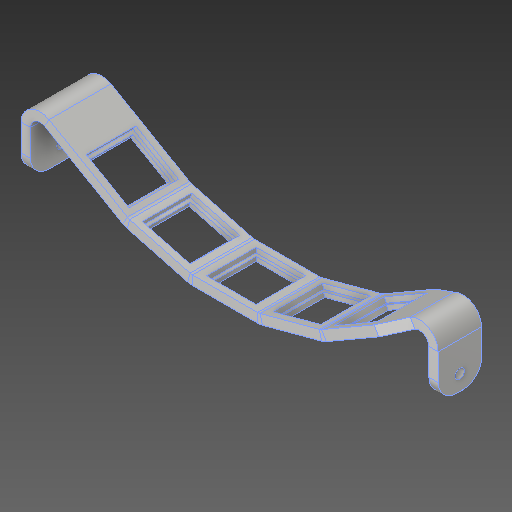
# Autodesk Inventor part: keyplate5
Saved by Autodesk Inventor 2018 (Build 220112000, 112)
## iProperties
Created: 2018-05-25
Part Number: keyplate5
Material: アルミニウム 6061
Document SubType Name: Sheet Metal
Designer: NaMACHAN
Density: 2.7 g/cm^3
Sheet Metal Rule: Al2mm
Appearance: アルミニウム - フラット
Mass: 16.9543 g
Surface Area: 65.7623 cm^2
Volume: 6.27936 cm^3
Author: NaMACHAN
Autodesk Inventor part; units mm, degrees
ref_plane "YZ Plane" through (0, 0, 0) normal (1, 0, 0) x (0, 1, 0)
ref_plane "XZ Plane" through (0, 0, 0) normal (0, 1, 0) x (-1, 0, 0)
ref_plane "XY Plane" through (0, 0, 0) normal (0, 0, 1) x (1, 0, 0)
sketch "スケッチ1" plane through (0, 0, 0) normal (0, 1, 0) x (-1, 0, 0)
  line L0 (-10.5, -10) -> (10.5, -10)
  line L1 (10.5, -10) -> (10.5, 10)
  line L2 (10.5, 10) -> (-10.5, 10)
  line L3 (-10.5, 10) -> (-10.5, -10)
  line L4 (-10.5, -10) -> (10.5, 10) construction
  line L5 (10.5, -10) -> (-10.5, 10) construction
  line L6 (-7, -7) -> (7, -7)
  line L7 (7, -7) -> (7, 7)
  line L8 (7, 7) -> (-7, 7)
  line L9 (-7, 7) -> (-7, -7)
  line L10 (-7, -7) -> (7, 7) construction
  line L11 (7, -7) -> (-7, 7) construction
  point P0 (0, 0)
  dimension "d0" = 21
  dimension "d1" = 20
  dimension "d2" = 14
  dimension "d3" = 14
  measures "d0" distance of L2.end L1.end
  measures "d1" distance of L1.end L0.end
  measures "d2" distance of L8.end L7.end
  measures "d3" distance of L7.end L6.end
extrude "プレート1" add sketch "スケッチ1" along normal blind 3
sketch "スケッチ2" plane through (-11.2765, 3.1022, 10) normal (-0.258819, -0.9659258, 0) x (0.9659258, -0.258819, 0)
  line L0 (0, -20) -> (0, 0)
  line L1 (0, 0) -> (-20.2101, 0)
  line L2 (-20.2101, 0) -> (-20.2101, -20)
  line L3 (-20.2101, -20) -> (0, -20)
  constraints: 6 end point, 1 horizontal, 1 perpendicular, 1 vertical
edge flange "フランジ1" height 21 angle 15 thickness 3 bend radius 3 thickness toward (-0.258819, -0.9659258, 0) relief straight relief width 3 relief depth 1.5 edges at (-10.5, 3, 0) wall of the first edge with corners at (-11.2765, 3.1022, -10) (-11.2765, 3.1022, 10) (-30.7979, 8.333, 10) (-30.7979, 8.333, -10)
bend "曲げ1"
corner "コーナー1"
sketch "スケッチ3" plane through (11.2765, 3.1022, -10) normal (0.258819, -0.9659258, 0) x (0.9659258, 0.258819, 0)
  line L0 (0, 20) -> (0, 0)
  line L1 (0, 0) -> (20.2101, 0)
  line L2 (20.2101, 0) -> (20.2101, 20)
  line L3 (20.2101, 20) -> (0, 20)
  constraints: 8 end point
edge flange "フランジ2" height 21 angle 15 thickness 3 bend radius 3 thickness toward (0.258819, -0.9659258, 0) relief straight relief width 3 relief depth 1.5 edges at (10.5, 3, 0) wall of the first edge with corners at (11.2765, 3.1022, 10) (11.2765, 3.1022, -10) (30.7979, 8.333, -10) (30.7979, 8.333, 10)
bend "曲げ2"
corner "コーナー2"
sketch "スケッチ6" plane through (-31.5214, 8.6327, 10) normal (-0.5, -0.8660254, 0) x (0.8660254, -0.5, 0)
  line L0 (0, -20) -> (0, 0)
  line L1 (0, 0) -> (-29.2101, 0)
  line L2 (-29.2101, 0) -> (-29.2101, -20)
  line L3 (-29.2101, -20) -> (0, -20)
  constraints: 6 end point, 1 horizontal, 1 perpendicular, 1 vertical
edge flange "フランジ5" height 30 angle 15 thickness 3 bend radius 3 thickness toward (-0.5, -0.8660254, 0) relief straight relief width 3 relief depth 1.5 edges at (-30.7979, 8.333, 0) wall of the first edge with corners at (-31.5214, 8.6327, -10) (-31.5214, 8.6327, 10) (-56.8181, 23.2377, 10) (-56.8181, 23.2377, -10)
bend "曲げ5"
corner "コーナー5"
sketch "スケッチ7" plane through (11.2765, 3.1022, 10) normal (-0.258819, 0.9659258, 0) x (0.9659258, 0.258819, 0)
  line L0 (3.2367, 17) -> (17.2367, 17)
  line L1 (17.2367, 17) -> (17.2367, 3)
  line L2 (17.2367, 3) -> (3.2367, 3)
  line L3 (3.2367, 3) -> (3.2367, 17)
  line L4 (3.2367, 17) -> (17.2367, 3) construction
  line L5 (17.2367, 17) -> (3.2367, 3) construction
  line L6 (20.2101, 0) -> (0, 0) projected
  line L7 (-0.7765, 20) -> (-0.7765, 0) projected
  point P0 (-11.6951, 10)
  point P1 (10.2367, 10)
  point P2 (10.2367, 10)
  point P3 (10.2367, 0)
  point P4 (20.4734, 0)
  point P5 (10.2367, 10)
  point P6 (-0.7765, 10)
  dimension "d55" = 14
  dimension "d56" = 14
  constraints: 12 end point, 5 midpoint, 2 parallel, 1 horizontal, 1 horizontal alignment, 1 perpendicular, 1 point on line, 1 vertical alignment
  measures "d55" distance of L1.end L2.end
  measures "d56" distance of L0.end L1.end
extrude "押し出し1" cut sketch "スケッチ7" against normal blind 10
sketch "スケッチ9" plane through (-11.2765, 3.1022, 10) normal (0.258819, 0.9659258, 0) x (0.9659258, -0.258819, 0)
  line L0 (-17.105, 17) -> (-3.105, 17)
  line L1 (-3.105, 17) -> (-3.105, 3)
  line L2 (-3.105, 3) -> (-17.105, 3)
  line L3 (-17.105, 3) -> (-17.105, 17)
  line L4 (-17.105, 17) -> (-3.105, 3) construction
  line L5 (-3.105, 17) -> (-17.105, 3) construction
  line L6 (-20.2101, 20) -> (-20.2101, 0) projected
  line L7 (-20.2101, 0) -> (0, 0) projected
  point P0 (11.6951, 10)
  point P1 (-10.105, 10)
  point P2 (-10.105, 10)
  point P3 (-20.2101, 10)
  point P4 (-10.105, 10)
  point P5 (-10.105, 0)
  dimension "d63" = 14
  dimension "d64" = 14
  constraints: 12 end point, 6 midpoint, 2 parallel, 1 horizontal, 1 horizontal alignment, 1 perpendicular, 1 vertical alignment
  measures "d63" distance of L1.end L2.end
  measures "d64" distance of L0.end L1.end
extrude "押し出し3" cut sketch "スケッチ9" against normal blind 10
sketch "スケッチ15" plane through (-31.5214, 8.6327, 10) normal (0.5, 0.8660254, 0) x (0.8660254, -0.5, 0)
  line L0 (-2.7008, 17) -> (-16.7008, 17)
  line L1 (-16.7008, 17) -> (-16.7008, 3)
  line L2 (-16.7008, 3) -> (-2.7008, 3)
  line L3 (-2.7008, 3) -> (-2.7008, 17)
  line L4 (-2.7008, 17) -> (-16.7008, 3) construction
  line L5 (-16.7008, 17) -> (-2.7008, 3) construction
  line L6 (0.7765, 20) -> (0.7765, 0) projected
  line L7 (-29.2101, 20) -> (0, 20) projected
  point P0 (31.6147, 10)
  point P1 (-9.7008, 10)
  point P2 (-9.7008, 10)
  point P3 (0.7765, 10)
  point P4 (-9.7008, 10)
  point P5 (-9.7008, 20)
  point P6 (-19.4016, 20)
  dimension "d93" = 14
  dimension "d94" = 14
  constraints: 12 end point, 5 midpoint, 2 parallel, 1 horizontal, 1 horizontal alignment, 1 perpendicular, 1 point on line, 1 vertical alignment
  measures "d93" distance of L2.end L1.end
  measures "d94" distance of L1.end L0.end
extrude "押し出し8" cut sketch "スケッチ15" against normal blind 10
sketch "スケッチ28" plane through (-62.8181, 18.0416, -10) normal (-1, 0, 0) x (0, -1, 0)
  line L0 (0, 20) -> (0, 0)
  line L1 (0, 0) -> (14.6077, 0)
  line L2 (14.6077, 0) -> (14.6077, 20)
  line L3 (14.6077, 20) -> (0, 20)
  constraints: 6 end point, 1 horizontal, 1 perpendicular, 1 vertical
edge flange "フランジ13" height 25 angle 120 thickness 3 bend radius 3 thickness toward (-1, 0, 0) relief straight relief width 3 relief depth 1.5 edges at (-58.3181, 20.6396, 0) wall of the first edge with corners at (-62.8181, 18.0416, 10) (-62.8181, 18.0416, -10) (-62.8181, 3.4339, -10) (-62.8181, 3.4339, 10)
bend "曲げ13"
corner "コーナー13"
ref_plane "作業平面1" through (30.7979, 8.333, 10) normal (-0.5, 0.8660254, 0) x (0, 0, -1)
sketch "スケッチ31" plane through (30.7979, 8.333, 10) normal (-0.5, 0.8660254, 0) x (0, 0, -1)
  line L0 (0, 0) -> (0, -20)
  line L1 (0, -20) -> (3, -30)
  line L2 (3, -30) -> (17, -30)
  line L3 (17, -30) -> (20, -20)
  line L4 (20, 0) -> (20, 19.5214)
  line L5 (20, -20) -> (20, 0)
  line L6 (0, 0) -> (20, 0)
  point P0 (10, 30.8383)
  point P1 (10, -30)
  point P2 (10, 0)
  dimension "d220" = 20
  dimension "d221" = 30
  dimension "d222" = 14
  measures "d220" distance of L0.start L0.end
  measures "d221" distance between parallel lines of L6 L2
  measures "d222" distance of L1.end L2.end
sheet face with bend "面2" sketch "スケッチ31" thickness 3 toward (0.5, -0.8660254, 0) bend radius 3 relief straight relief width 3 relief depth 1.5
bend "曲げ15"
sketch "スケッチ32" plane through (30.7979, 8.333, 10) normal (-0.5, 0.8660254, 0) x (0.8660254, 0.5, 0)
  line L0 (3.895, 3) -> (17.895, 3)
  line L1 (17.895, 3) -> (17.895, 17)
  line L2 (17.895, 17) -> (3.895, 17)
  line L3 (3.895, 17) -> (3.895, 3)
  line L4 (3.895, 3) -> (17.895, 17) construction
  line L5 (17.895, 3) -> (3.895, 17) construction
  line L6 (-0.3815, 0) -> (-0.3815, 20) projected
  line L7 (0.395, 0) -> (0.395, 20) projected
  point P0 (-30.8383, 10)
  point P1 (10.895, 10)
  point P2 (10.895, 10)
  point P3 (-0.3815, 10)
  dimension "d228" = 14
  dimension "d229" = 14
  dimension "d230" = 10.5
  constraints: 12 end point, 4 midpoint, 2 parallel, 1 horizontal, 1 horizontal alignment, 1 perpendicular
  measures "d228" distance of L2.end L1.end
  measures "d229" distance of L1.end L0.end
  measures "d230" distance from line of L7 point (10.895, 10)
extrude "押し出し13" cut sketch "スケッチ32" against normal blind 10
sketch "スケッチ33" plane through (62.7787, 18.1368, 7) normal (1, 0, 0) x (0, 1, 0)
  line L0 (0, -14) -> (0, 0)
  line L1 (0, 0) -> (-14.6077, 0)
  line L2 (-14.6077, 0) -> (-14.6077, -14)
  line L3 (-14.6077, -14) -> (0, -14)
  constraints: 6 end point, 1 horizontal, 1 perpendicular, 1 vertical
edge flange "フランジ15" height 25 angle 120 thickness 3 bend radius 3 thickness toward (1, 0, 0) relief straight relief width 3 relief depth 1.5 edges at (58.2787, 20.7349, 0) wall of the first edge with corners at (62.7787, 18.1368, -7) (62.7787, 18.1368, 7) (62.7787, 3.5291, 7) (62.7787, 3.5291, -7)
bend "曲げ16"
corner "コーナー15"
sketch "スケッチ34" plane through (65.7787, 3.5291, 7) normal (1, 0, 0) x (0, 0, -1)
  line L0 (14, 0) -> (0, 0) projected
  point P0 (7, -3.5291)
  point P1 (7, 5)
  dimension "d243" = 5
  constraints: 1 vertical alignment
  measures "d243" distance from line of L0 point (7, 5)
hole "穴3" at (65.7787, 8.5291, 0) direction (-1, 0, 0) diameter 3 depth 3 tip angle 118
sketch "スケッチ35" plane through (-65.8181, 3.4339, -10) normal (-1, 0, 0) x (0, 0, 1)
  circle A0 centre (10, 5.0953) radius 1.5 projected
  point P0 (10, -3.4339)
  constraints: 1 coincident
hole "穴4" at (-65.8181, 8.5291, 0) direction (1, 0, 0) diameter 3 depth 3 tip angle 118
sketch "スケッチ36" plane through (-31.5214, 8.6327, 10) normal (0.5, 0.8660254, 0) x (0.8660254, -0.5, 0)
  line L0 (-1.7008, 18) -> (-17.7008, 18)
  line L1 (-17.7008, 18) -> (-17.7008, 2)
  line L2 (-17.7008, 2) -> (-1.7008, 2)
  line L3 (-1.7008, 2) -> (-1.7008, 18)
  line L4 (-1.7008, 18) -> (-17.7008, 2) construction
  line L5 (-17.7008, 18) -> (-1.7008, 2) construction
  line L6 (-16.7008, 3) -> (-16.7008, 17) projected
  line L7 (-16.7008, 17) -> (-2.7008, 17) projected
  point P0 (31.6147, 10)
  point P1 (-9.7008, 10)
  point P2 (-9.7008, 10)
  point P3 (-16.7008, 10)
  point P4 (-9.7008, 10)
  point P5 (-9.7008, 17)
  dimension "d258" = 16
  dimension "d259" = 16
  constraints: 12 end point, 6 midpoint, 2 parallel, 1 horizontal, 1 horizontal alignment, 1 perpendicular, 1 vertical alignment
  measures "d258" distance of L2.end L1.end
  measures "d259" distance of L1.end L0.end
extrude "押し出し14" cut sketch "スケッチ36" against normal blind 1.6
sketch "スケッチ37" plane through (-11.2765, 3.1022, 10) normal (0.258819, 0.9659258, 0) x (0.9659258, -0.258819, 0)
  line L0 (-2.105, 18) -> (-18.105, 18)
  line L1 (-18.105, 18) -> (-18.105, 2)
  line L2 (-18.105, 2) -> (-2.105, 2)
  line L3 (-2.105, 2) -> (-2.105, 18)
  line L4 (-2.105, 18) -> (-18.105, 2) construction
  line L5 (-18.105, 18) -> (-2.105, 2) construction
  line L6 (-17.105, 3) -> (-17.105, 17) projected
  line L7 (-17.105, 17) -> (-3.105, 17) projected
  point P0 (11.6951, 10)
  point P1 (-10.105, 10)
  point P2 (-10.105, 10)
  point P3 (-17.105, 10)
  point P4 (-10.105, 10)
  point P5 (-10.105, 17)
  dimension "d262" = 16
  dimension "d263" = 16
  constraints: 12 end point, 6 midpoint, 2 parallel, 1 horizontal, 1 horizontal alignment, 1 perpendicular, 1 vertical alignment
  measures "d262" distance of L2.end L1.end
  measures "d263" distance of L1.end L0.end
extrude "押し出し15" cut sketch "スケッチ37" against normal blind 1.6
sketch "スケッチ38" plane through (0, 3, 0) normal (0, 1, 0) x (1, 0, 0)
  line L0 (8, 8) -> (-8, 8)
  line L1 (-8, 8) -> (-8, -8)
  line L2 (-8, -8) -> (8, -8)
  line L3 (8, -8) -> (8, 8)
  line L4 (8, 8) -> (-8, -8) construction
  line L5 (-8, 8) -> (8, -8) construction
  point P0 (0, 0)
  dimension "d266" = 16
  dimension "d267" = 16
  constraints: 12 end point, 2 midpoint, 2 parallel, 1 horizontal, 1 perpendicular
  measures "d266" distance of L2.end L1.end
  measures "d267" distance of L1.end L0.end
extrude "押し出し16" cut sketch "スケッチ38" against normal blind 1.6
sketch "スケッチ39" plane through (11.2765, 3.1022, 10) normal (-0.258819, 0.9659258, 0) x (0.9659258, 0.258819, 0)
  line L0 (18.2367, 18) -> (2.2367, 18)
  line L1 (2.2367, 18) -> (2.2367, 2)
  line L2 (2.2367, 2) -> (18.2367, 2)
  line L3 (18.2367, 2) -> (18.2367, 18)
  line L4 (18.2367, 18) -> (2.2367, 2) construction
  line L5 (2.2367, 18) -> (18.2367, 2) construction
  line L6 (3.2367, 3) -> (3.2367, 17) projected
  line L7 (3.2367, 17) -> (17.2367, 17) projected
  point P0 (-11.6951, 10)
  point P1 (10.2367, 10)
  point P2 (10.2367, 10)
  point P3 (3.2367, 10)
  point P4 (10.2367, 10)
  point P5 (10.2367, 17)
  dimension "d270" = 16
  dimension "d271" = 16
  constraints: 12 end point, 6 midpoint, 2 parallel, 1 horizontal, 1 horizontal alignment, 1 perpendicular, 1 vertical alignment
  measures "d270" distance of L2.end L1.end
  measures "d271" distance of L1.end L0.end
extrude "押し出し17" cut sketch "スケッチ39" against normal blind 1.6
sketch "スケッチ40" plane through (30.7979, 8.333, 10) normal (-0.5, 0.8660254, 0) x (0.8660254, 0.5, 0)
  point P0 (-30.8383, 10)
sketch "スケッチ41" plane through (30.7979, 8.333, 10) normal (-0.5, 0.8660254, 0) x (0.8660254, 0.5, 0)
  line L0 (18.895, 18) -> (2.895, 18)
  line L1 (2.895, 18) -> (2.895, 2)
  line L2 (2.895, 2) -> (18.895, 2)
  line L3 (18.895, 2) -> (18.895, 18)
  line L4 (18.895, 18) -> (2.895, 2) construction
  line L5 (2.895, 18) -> (18.895, 2) construction
  line L6 (3.895, 17) -> (17.895, 17) projected
  line L7 (3.895, 3) -> (3.895, 17) projected
  point P0 (-30.8383, 10)
  point P1 (10.895, 10)
  point P2 (10.895, 10)
  point P3 (10.895, 17)
  point P4 (10.895, 10)
  point P5 (3.895, 10)
  dimension "d274" = 16
  dimension "d275" = 16
  constraints: 12 end point, 6 midpoint, 2 parallel, 1 horizontal, 1 horizontal alignment, 1 perpendicular, 1 vertical alignment
  measures "d274" distance of L2.end L1.end
  measures "d275" distance of L1.end L0.end
extrude "押し出し18" cut sketch "スケッチ41" against normal blind 1.6
fillet "コーナーR2" radius 6 4 edges at (64.2787, 3.5291, 7) (64.2787, 3.5291, -7) (-64.3181, 3.4339, 10) (-64.3181, 3.4339, -10)
equation "\"d249\" = Thickness"
equation "\"d256\" = Thickness"
equation "\"d4\" = Thickness"
equation "\"d5\" = BendReliefWidth"
equation "\"d6\" = BendReliefDepth"
equation "\"d7\" = MinimumRemnant"
equation "\"d8\" = TransitionRadius"
equation "\"d11\" = BendRadius"
equation "\"d12\" = CornerReliefSize"
equation "\"d13\" = GapSize"
equation "\"d14\" = JacobiRadiusSize"
equation "\"d15\" = BendReliefWidth"
equation "\"d16\" = BendReliefDepth"
equation "\"d17\" = MinimumRemnant"
equation "\"d18\" = TransitionRadius"
equation "\"d21\" = BendRadius"
equation "\"d22\" = CornerReliefSize"
equation "\"d23\" = GapSize"
equation "\"d24\" = JacobiRadiusSize"
equation "\"d45\" = BendReliefWidth"
equation "\"d46\" = BendReliefDepth"
equation "\"d47\" = MinimumRemnant"
equation "\"d48\" = TransitionRadius"
equation "\"d51\" = BendRadius"
equation "\"d52\" = CornerReliefSize"
equation "\"d53\" = GapSize"
equation "\"d54\" = JacobiRadiusSize"
equation "\"d191\" = BendReliefWidth"
equation "\"d192\" = BendReliefDepth"
equation "\"d193\" = MinimumRemnant"
equation "\"d194\" = TransitionRadius"
equation "\"d197\" = BendRadius"
equation "\"d198\" = CornerReliefSize"
equation "\"d199\" = GapSize"
equation "\"d200\" = JacobiRadiusSize"
equation "\"d223\" = BendRadius"
equation "\"d224\" = BendReliefWidth"
equation "\"d226\" = MinimumRemnant"
equation "\"d225\" = BendReliefDepth"
equation "\"d227\" = TransitionRadius"
equation "\"d233\" = BendReliefWidth"
equation "\"d234\" = BendReliefDepth"
equation "\"d235\" = MinimumRemnant"
equation "\"d236\" = TransitionRadius"
equation "\"d239\" = BendRadius"
equation "\"d240\" = CornerReliefSize"
equation "\"d241\" = GapSize"
equation "\"d242\" = JacobiRadiusSize"
equation "\"BendRadius\" = Thickness"
equation "\"BendReliefWidth\" = Thickness"
equation "\"BendReliefDepth\" = 0.5 * Thickness"
equation "\"CornerReliefSize\" = 4 * Thickness"
equation "\"MinimumRemnant\" = 2 * Thickness"
equation "\"TransitionRadius\" = BendRadius"
equation "\"JacobiRadiusSize\" = BendRadius"
equation "\"GapSize\" = Thickness"
equation "\"Thickness\" = 3"
